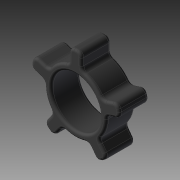
# Autodesk Inventor part: 2102_Tx_Coil_Fins_V1
Saved by Autodesk Inventor 2021 (Build 250183000, 183)
## iProperties
Created: 2022-06-20
Part Number: 2102_Tx_Coil_Fins_V1
Material: Generic
Document SubType Name: Modeling
Designer: Eli
Density: 1 g/cm^3
Appearance: Default
Author: Eli
Autodesk Inventor part; units mm, degrees
ref_plane "YZ Plane" through (0, 0, 0) normal (1, 0, 0) x (0, 1, 0)
ref_plane "XZ Plane" through (0, 0, 0) normal (0, 1, 0) x (-1, 0, 0)
ref_plane "XY Plane" through (0, 0, 0) normal (0, 0, 1) x (1, 0, 0)
sketch "Sketch1" plane through (0, 0, 0) normal (0, 0, 1) x (1, 0, 0)
  circle A0 centre (0, 0) radius 10
  circle A1 centre (0, 0) radius 12.5
  circle A2 centre (0, 0) radius 19 construction
  dimension "d0" = 20
  dimension "d1" = 2.5
  dimension "d2" = 38
  constraints: 3 centre point, 2 coincident
  measures "d0" diameter of A0
  measures "d1" radial gap between concentric circles of A0 A1
  measures "d2" diameter of A2
extrude "Extrusion1" add sketch "Sketch1" along normal blind 12
sketch "Sketch2" plane through (0, 0, 12) normal (0, 0, 1) x (1, 0, 0)
  circle A0 centre (0, 0) radius 12.5 projected
  circle A1 centre (0, 0) radius 12.5 projected
  circle A2 centre (0, 0) radius 18.65
  line L0 (-2.5, 18.65) -> (2.5, 18.65)
  line L1 (2.5, 18.65) -> (2.5, 0.7124)
  line L2 (2.5, 0.7124) -> (-2.5, 0.7124)
  line L3 (-2.5, 0.7124) -> (-2.5, 18.65)
  point P0 (0, 18.65)
  point P1 (-2.5, 18.4817)
  point P2 (-2.5, 12.2474)
  point P3 (2.5, 12.2474)
  point P4 (2.5, 18.4817)
  dimension "d5" = 37.3
  dimension "d6" = 5
  constraints: 8 end point, 2 parallel, 1 centre point, 1 coincident, 1 horizontal, 1 midpoint, 1 perpendicular, 1 tangent, 1 vertical alignment
  measures "d5" diameter of A2
  measures "d6" distance between parallel lines of L1 L3
extrude "Extrusion2" add sketch "Sketch2" against normal up to surface (12 mm away) contours A0 L3 A2 L1 picked at (0, 14.5312)
fillet "Fillet1" radius 2 4 edges at (2.5, 12.2474, 6) (-2.5, 12.2474, 6) (-2.5, 18.4817, 6) (2.5, 18.4817, 6)
pattern_circular "Circular Pattern1" count 5 over 360 about axis through (0, 0, 0) along (0, 0, 1) of "Extrusion2", "Fillet1"
fillet "Fillet2" radius 1 27 edges at (2.5, 15.2133, 12) (0, 18.65, 12) (-2.5, 15.2133, 12) (-7.3473, 10.1127, 12) (-13.6961, 7.0788, 12) (-17.7372, 5.7632, 12) (-15.2412, 2.3235, 12) (-11.8882, -3.8627, 12) (-10.9647, -10.8383, 12) (-10.9622, -15.0882, 12) (-6.9196, -13.7773, 12) (0, -12.5, 12) (6.9196, -13.7773, 12) (10.9622, -15.0882, 12) (10.9647, -10.8383, 12) (11.8882, -3.8627, 12) (15.2412, 2.3235, 12) (17.7372, 5.7632, 12) (13.6961, 7.0788, 12) (7.3473, 10.1127, 12) (-7.3473, 10.1127, 0) (-11.8882, -3.8627, 0) (0, -12.5, 0) (11.8882, -3.8627, 0) (7.3473, 10.1127, 0) (-10, 0, 12) (-10, 0, 0)
body "Solid1"
